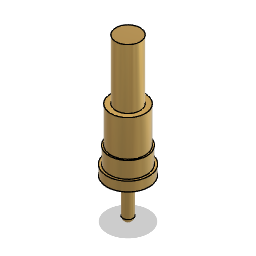
baseline_pcb_only (Autodesk Fusion 360 archive; units mm, degrees)
design "2906-4-15-20-75-14-11-0"
Autodesk Fusion 360 part; units mm, degrees
imported_body "Base Feature1" makes body 1
sketch "thru_hole_mount" plane through (0, 0, 0) normal (0, 1, 0) x (1, 0, 0)
  circle A0 centre (0, 0) radius 0.215
  dimension "d1" = 0.43
  constraint coincident A0.centre origin
  measures "d1" diameter of A0
extrude "Extrude1" add sketch "thru_hole_mount" along normal blind 1.75 separate body makes body 2
sketch "pcb_flange" plane through (0, 1.75, 0) normal (0, 1, 0) x (-1, 0, 0)
  circle A0 centre (0, 0) radius 0.215
  circle A1 centre (0, 0) radius 0.915
  dimension "d4" = 1.83
  constraint coincident A0.centre A1.centre
  measures "d4" diameter of A1
extrude "Extrude2" add sketch "pcb_flange" along normal blind 0.41 contours A0 | A1 bodies 2
sketch "above_flange" plane through (0, 2.16, 0) normal (0, 1, 0) x (-1, 0, 0)
  circle A0 centre (0, 0) radius 0.915
  circle A1 centre (0, 0) radius 0.815
  dimension "d7" = 1.63
  constraint concentric A0 A1
  measures "d7" diameter of A1
extrude "Extrude3" add sketch "above_flange" along normal blind 0.71 contours A1 bodies 2
sketch "pin_sheath" plane through (0, 2.87, 0) normal (0, 1, 0) x (-1, 0, 0)
  circle A0 centre (0, 0) radius 0.815
  circle A1 centre (0, 0) radius 0.75
  dimension "d10" = 1.5
  constraint concentric A0 A1
  measures "d10" diameter of A1
extrude "Extrude4" add sketch "pin_sheath" along normal blind 1.57 contours A1 bodies 2
sketch "Sketch5" plane through (0, 4.44, 0) normal (0, 1, 0) x (-1, 0, 0)
  circle A0 centre (0, 0) radius 0.75
  circle A1 centre (0, 0) radius 0.53
  dimension "d13" = 1.06
  constraint coincident A0.centre A1.centre
  measures "d13" diameter of A1
extrude "Extrude5" add sketch "Sketch5" along normal blind 2.6 contours A1 bodies 2
move_body "Move1" bodies 2 to x (1, 0, 0) y (0, 1, 0) z (0, 0, 1) at (-11.0246, -5.2641, -12.4361)
fillet "Fillet1" radius 0.2099 1 faces at (-10.8444, -5.2641, -12.4233) on bodies 2
hidden bodies 1
equation "d11 = 2.69 mm - 0.71 mm - 0.41 mm"
equation "d14 = 5.99 mm - 2.69 mm - 0.7 mm"
named bodies: "0906-4-15-20-75-14-11-0 (Optimal Height)", "2906-4-15-20-75-14-11-0"
